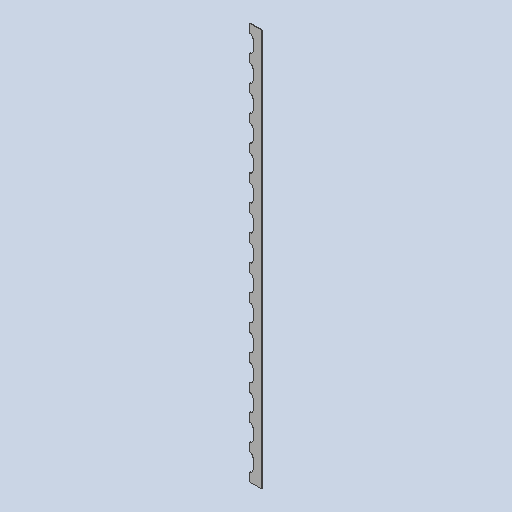
# Autodesk Inventor part: BSH 045 stringer partition 5
Saved by Autodesk Inventor 2025 (Build 290162010, 162A)
## iProperties
Created: 2024-07-23
Part Number: BSH 045 stringer partition 5
Material: 09g2s
Document SubType Name: Sheet Metal
Designer: admin
Density: 7.85 g/cm^3
Sheet Metal Rule: AISI304 3mm Die 32
Sheet Metal Width: 0,000 mm
Sheet Metal Length: 0,000 mm
Sheet Metal Area: 0,000 mm^2
Appearance: Default
Author: admin
Autodesk Inventor part; units mm, degrees
ref_plane "YZ Plane" through (0, 0, 0) normal (1, 0, 0) x (0, 1, 0)
ref_plane "XZ Plane" through (0, 0, 0) normal (0, 1, 0) x (-1, 0, 0)
ref_plane "XY Plane" through (0, 0, 0) normal (0, 0, 1) x (1, 0, 0)
sketch "Sketch6" plane through (0, 0, 0) normal (0, 1, 0) x (-1, 0, 0)
  line L0 (0, -1150) -> (-70.4709, -1150)
  line L1 (-70.4709, -1150) -> (-70.4709, 1150)
  line L2 (-70.4709, 1150) -> (0, 1150)
  line L3 (0, 1150) -> (0, -1150)
  point P0 (0, 0)
  point P1 (0, 0)
  dimension "d26" = 70.4709
  dimension "d27" = 2300
  measures "d26" distance of L1.end L2.end
  measures "d27" distance of L0.end L1.end
extrude "Plate4" add sketch "Sketch6" along normal blind 3
sketch "Sketch7" plane through (0, 0, 0) normal (0, -1, 0) x (1, 0, 0)
  line L0 (0, 1150) -> (70.4709, 1150) projected
  line L1 (0, -1150) -> (0, 1150) projected
  line L2 (70.4709, -1150) -> (0, -1150) projected
  line L3 (70.4709, 1150) -> (70.4709, -1150) projected
  line L4 (20, -30) -> (20, 30)
  arc A0 (0, -50) -> (20, -30) centre (0, -30) ccw
  arc A1 (20, 30) -> (0, 50) centre (0, 30) ccw
  point P0 (0, 0)
  point P1 (20, 0)
  point P2 (0, 0)
  dimension "d37" = 20
  dimension "d38" = 100
  constraints: 4 point on circle, 4 point on line, 2 centre point, 2 end point, 2 midpoint, 2 tangent, 1 horizontal alignment, 1 vertical
  measures "d37" distance between parallel lines of L1 L4
  measures "d38" distance of A1.end A0.start
extrude "Extrusion2" cut sketch "Sketch7" against normal through all contours A1 L4 A0 L1
pattern_linear "Rectangular Pattern2" count 15 spacing 150 along (0, 0, 1) of "Extrusion2" first direction both ways yes
equation "\"d26\" = Stringer3_deep"
equation "\"d28\" = Thickness"
equation "\"BendReliefWidth\" = Thickness"
equation "\"BendReliefDepth\" = 0.5 * Thickness"
equation "\"CornerReliefSize\" = 4 * Thickness"
equation "\"MinimumRemnant\" = 2 * Thickness"
equation "\"TransitionRadius\" = BendRadius"
equation "\"JacobiRadiusSize\" = BendRadius"
equation "\"GapSize\" = Thickness"
equation "\"Stringer3_deep\" = 70.470938"
equation "\"Thickness\" = 3"
equation "\"BendRadius\" = 5"
body "Solid2"
